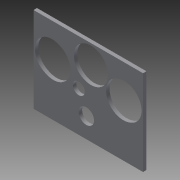
# Autodesk Inventor part: OutlineSketch1
Saved by Autodesk Inventor 2013 (Build 170138000, 138)
## iProperties
Created: 2013-06-03
Part Number: OutlineSketch1
Material: Generic
Document SubType Name: Modeling
Designer: mvarma
Density: 1 g/cm^3
Author: mvarma
Autodesk Inventor part; units mm, degrees
ref_plane "YZ Plane" through (0, 0, 0) normal (1, 0, 0) x (0, 1, 0)
ref_plane "XZ Plane" through (0, 0, 0) normal (0, 1, 0) x (-1, 0, 0)
ref_plane "XY Plane" through (0, 0, 0) normal (0, 0, 1) x (1, 0, 0)
sketch "Sketch1" plane through (0, 0, 0) normal (0, 0, 1) x (1, 0, 0)
  line L0 (0, 0) -> (304.8, 0) construction
  line L1 (304.8, 0) -> (304.8, 50.8) construction
  line L2 (304.8, 50.8) -> (0, 50.8) construction
  line L3 (0, 50.8) -> (0, 0) construction
  circle A0 centre (152.4, 25.4) radius 14.2875
  circle A1 centre (152.4, 25.4) radius 30.48 construction
  circle A2 centre (152.4, 25.4) radius 22.225 construction
  line L4 (152.4, 25.4) -> (138.508178, 62.969727) construction
  circle A3 centre (138.508178, 62.969727) radius 9.525 construction
  circle A4 centre (138.508178, 62.969727) radius 17.78 construction
  circle A5 centre (89.971088, 85.09) radius 31.75 construction
  circle A6 centre (160.978478, 111.345767) radius 31.75
  circle A7 centre (221.970096, 85.09) radius 31.75 construction
  line L5 (0, 50.8) -> (0, 53.34) construction
  line L6 (0, 53.34) -> (304.8, 53.34) construction
  line L7 (304.8, 53.34) -> (304.8, 50.8) construction
  circle A8 centre (138.508178, 62.969727) radius 21.59 construction
  circle A9 centre (152.4, 25.4) radius 46.99 construction
  circle A10 centre (152.4, 25.4) radius 50.8 construction
  arc A11 (84.94082, 79.326416) -> (90.918413, 92.681118) centre (89.971088, 85.09) ccw construction
  circle A12 centre (160.978478, 111.345767) radius 7.65 construction
  arc A13 (221.694578, 92.735037) -> (225.517168, 78.312037) centre (221.970096, 85.09) ccw construction
  circle A14 centre (160.978478, 111.345767) radius 9.1 construction
  circle A15 centre (138.508178, 62.969727) radius 22.9 construction
  line L8 (84.94082, 79.326416) -> (123.450252, 45.716644) construction
  line L9 (168.548316, 110.241211) -> (161.168218, 59.663279) construction
  line L10 (90.918413, 92.681118) -> (89.971088, 85.09) construction
  line L11 (89.971088, 85.09) -> (84.94082, 79.326416) construction
  circle A16 centre (126.19198, 96.27826) radius 3.175 construction
  circle A17 centre (126.19198, 96.27826) radius 7.9375 construction
  line L12 (90.918413, 92.681118) -> (125.209053, 88.401855) construction
  line L13 (132.062639, 90.936044) -> (155.320457, 116.494485) construction
  line L14 (155.320457, 116.494485) -> (160.978478, 111.345767) construction
  line L15 (168.548316, 110.241211) -> (160.978478, 111.345767) construction
  line L16 (138.508178, 62.969727) -> (126.19198, 96.27826) construction
  line L17 (89.971088, 85.09) -> (160.978478, 111.345767) construction
  line L18 (152.4, 25.4) -> (89.971088, 85.09) construction
  line L19 (152.4, 25.4) -> (160.978478, 111.345767) construction
  circle A18 centre (126.19198, 96.27826) radius 9.2075 construction
  circle A19 centre (126.19198, 96.27826) radius 6.1595 construction
  arc A20 (90.918413, 92.681118) -> (84.94082, 79.326416) centre (89.971088, 85.09) ccw construction
  circle A21 centre (160.978478, 111.345767) radius 25.4 construction
  circle A22 centre (221.970096, 85.09) radius 25.4 construction
  line L20 (102.942353, 114.069454) -> (76.999823, 56.110546) construction
  circle A23 centre (89.971088, 85.09) radius 25.4 construction
  line L21 (213.836088, 115.780396) -> (230.104105, 54.399604) construction
  line L22 (54.411088, 146.905767) -> (257.611088, 146.905767)
  line L23 (257.611088, 146.905767) -> (257.611088, -11.844233)
  line L24 (257.611088, -11.844233) -> (54.411088, -11.844233)
  line L25 (54.411088, -11.844233) -> (54.411088, 146.905767)
  circle A24 centre (138.508178, 62.969727) radius 11.1125
  arc A25 (225.312875, 75.445533) -> (221.093638, 95.322667) centre (223.203256, 85.3841) ccw construction
  line L26 (220.753147, 84.734737) -> (228.477303, 60.537683) construction
  line L27 (223.203256, 85.3841) -> (228.477303, 60.537683) construction
  line L28 (220.753147, 84.734737) -> (213.028991, 108.931791) construction
  line L29 (223.203256, 85.3841) -> (217.92921, 110.230517) construction
  arc A26 (212.304851, 111.200264) -> (213.75313, 106.663317) centre (213.028991, 108.931791) ccw construction
  arc A27 (218.423652, 107.901165) -> (217.434768, 112.559869) centre (217.92921, 110.230517) ccw construction
  arc A28 (218.423652, 107.901165) -> (213.75313, 106.663317) centre (228.477303, 60.537683) ccw construction
  arc A29 (217.434768, 112.559869) -> (212.304851, 111.200264) centre (228.477303, 60.537683) ccw construction
  line L30 (213.028991, 108.931791) -> (212.304851, 111.200264) construction
  line L31 (217.92921, 110.230517) -> (217.434768, 112.559869) construction
  arc A30 (221.093638, 95.322667) -> (217.663484, 94.413558) centre (228.477303, 60.537683) ccw construction
  arc A31 (225.312875, 75.445533) -> (223.842809, 75.055915) centre (228.477303, 60.537683) ccw construction
  line L32 (102.635769, 107.180274) -> (91.114923, 84.543355) construction
  line L33 (79.594076, 61.906436) -> (88.801403, 85.578892) construction
  arc A32 (98.871917, 111.470639) -> (97.145543, 107.032054) centre (98.00873, 109.251347) ccw construction
  arc A33 (101.55569, 105.058063) -> (103.715849, 109.302485) centre (102.635769, 107.180274) ccw construction
  arc A34 (101.55569, 105.058063) -> (97.145543, 107.032054) centre (79.594076, 61.906436) ccw construction
  line L34 (98.00873, 109.251347) -> (98.871917, 111.470639) construction
  line L35 (102.635769, 107.180274) -> (103.715849, 109.302485) construction
  arc A35 (103.715849, 109.302485) -> (98.871917, 111.470639) centre (79.594076, 61.906436) ccw construction
  arc A36 (217.663484, 94.413558) -> (223.842809, 75.055915) centre (220.753147, 84.734737) ccw construction
  arc A37 (86.506584, 75.488588) -> (95.723261, 93.598123) centre (91.114923, 84.543355) ccw construction
  line L36 (88.801403, 85.578892) -> (98.00873, 109.251347) construction
  line L37 (91.114923, 84.543355) -> (79.594076, 61.906436) construction
  arc A38 (86.506584, 75.488588) -> (85.118472, 76.10991) centre (79.594076, 61.906436) ccw construction
  arc A39 (95.723261, 93.598123) -> (92.484334, 95.047874) centre (79.594076, 61.906436) ccw construction
  arc A40 (92.484334, 95.047874) -> (85.118472, 76.10991) centre (88.801403, 85.578892) ccw construction
  line L38 (160.978478, 111.345767) -> (138.015112, 122.201357) construction
  line L39 (160.978478, 111.345767) -> (183.941843, 100.490177) construction
  circle A41 centre (138.508178, 62.969727) radius 26.75 construction
  line L40 (221.694578, 92.735037) -> (137.544764, 89.702373) construction
  line L41 (225.517168, 78.312037) -> (150.911337, 39.269007) construction
  line L42 (221.970096, 85.09) -> (221.694578, 92.735037) construction
  line L43 (221.970096, 85.09) -> (225.517168, 78.312037) construction
  line L44 (138.508178, 62.969727) -> (137.544764, 89.702373) construction
  line L45 (138.508178, 62.969727) -> (150.911337, 39.269007) construction
  arc A42 (225.517168, 78.312037) -> (221.694578, 92.735037) centre (221.970096, 85.09) ccw construction
  arc A43 (225.517168, 78.312037) -> (224.776319, 77.973286) centre (221.970096, 85.09) ccw construction
  line L46 (138.508178, 62.969727) -> (221.970096, 85.09) construction
  circle A44 centre (88.801403, 85.578892) radius 31.75
  circle A45 centre (91.114923, 84.543355) radius 31.75
  line L47 (98.871917, 111.470639) -> (100.310562, 115.16946) construction
  line L48 (103.715849, 109.302485) -> (105.515981, 112.839504) construction
  arc A46 (105.515981, 112.839504) -> (100.310562, 115.16946) centre (79.594076, 61.906436) ccw
  circle A47 centre (220.753147, 84.734737) radius 31.75
  circle A48 centre (223.203256, 85.3841) radius 31.75
  line L49 (212.304851, 111.200264) -> (211.097951, 114.981054) construction
  line L50 (217.434768, 112.559869) -> (216.610698, 116.442121) construction
  arc A49 (216.610698, 116.442121) -> (211.097951, 114.981054) centre (228.477303, 60.537683) ccw
  point P0 (215.46289, 109.642317)
  point P1 (100.3481, 108.273564)
  dimension "d114" = 63.5
  dimension "d115" = 63.5
  dimension "d122" = 63.5
  dimension "d123" = 63.5
  dimension "d1" = 50.8
  dimension "d2" = 28.575
  dimension "d3" = 25.4
  dimension "d4" = 152.4
  dimension "d7" = 60.96
  dimension "d8" = 44.45
  dimension "d9" = 19.05
  dimension "d10" = 35.56
  dimension "d11" = 40.0558
  dimension "d12" = 63.5
  dimension "d13" = 63.5
  dimension "d14" = 63.5
  dimension "d15" = 2.54
  dimension "d16" = 304.8
  dimension "d17" = 43.18
  dimension "d18" = 93.98
  dimension "d19" = 101.6
  dimension "d21" = 15.3
  dimension "d22" = 15.3
  dimension "d24" = 18.2
  dimension "d29" = 45.8
  dimension "d30" = 146
  dimension "d31" = 6.35
  dimension "d32" = 15.875
  dimension "d33" = 146
  dimension "d35" = 18.415
  dimension "d37" = 12.319
  dimension "d40" = 50.8
  dimension "d41" = 50.8
  dimension "d42" = 17
  dimension "d43" = 17
  dimension "d44" = 50.8
  dimension "d53" = 203.2
  dimension "d54" = 158.75
  dimension "d55" = 35.56
  dimension "d56" = 35.56
  dimension "d57" = 22.225
  dimension "d67" = 25.4
  dimension "d68" = 25.4
  dimension "d69" = 2.86
  dimension "d70" = 25.4
  dimension "d71" = 25.4
  dimension "d72" = 4.7625
  dimension "d75" = 2.86
  dimension "d80" = 4.7625
  dimension "d82" = 4.7625
  dimension "d83" = 50.8
  dimension "d84" = 50.8
  dimension "d85" = 10.16
  dimension "d97" = 48.41875
  dimension "d99" = 20.32
  dimension "d101" = 25.4
  dimension "d102" = 25.4
  dimension "d103" = 10.16
  dimension "d105" = 17
  dimension "d106" = 17
  dimension "d107" = 53.5
  dimension "d108" = 154.44
  dimension "d109" = 7.65
  dimension "d111" = 86.34349
  dimension "d112" = 12.7801
  dimension "d113" = 12.7801
  dimension "d116" = 57.15
  constraints: 104 end point, 67 point on circle, 46 centre point, 38 coincident, 18 tangent, 14 collinear, 14 point on line, 9 perpendicular, 7 parallel, 2 horizontal, 2 midpoint, 1 equal radius, 15 other
  measures "d1" distance of L1.end L0.end
  measures "d2" diameter of A0
  measures "d3" distance from line of L0 A0.centre
  measures "d4" distance from line of L3 A0.centre
  measures "d7" diameter of A1
  measures "d8" diameter of A2
  measures "d9" diameter of A3
  measures "d10" diameter of A4
  measures "d11" distance of L4.start L4.end
  measures "d12" diameter of A5
  measures "d13" diameter of A6
  measures "d14" diameter of A7
  measures "d15" distance of L2.end L5.end
  measures "d16" distance of L0.end L0.start
  measures "d17" diameter of A8
  measures "d18" diameter of A9
  measures "d19" diameter of A10
  measures "d21" diameter of A11
  measures "d22" diameter of A12
  measures "d24" diameter of A14
  measures "d29" diameter of A15
  measures "d30" angle of L11 L10
  measures "d31" diameter of A16
  measures "d32" diameter of A17
  measures "d33" angle of L15 L14
  measures "d35" diameter of A18
  measures "d37" diameter of A19
  measures "d40" diameter of A21
  measures "d41" diameter of A22
  measures "d42" angle of L10 L20
  measures "d43" angle of L11 L20
  measures "d44" diameter of A23
  measures "d53" distance of L23.end L24.end
  measures "d54" distance of L22.end L23.end
  measures "d55" distance from line of L25 A5.centre
  measures "d56" distance from line of L22 A6.centre
  measures "d57" diameter of A24
  measures "d67" distance of L26.start L26.end
  measures "d68" distance of L27.start L26.end
  measures "d69" angle of L21 L26
  measures "d70" distance of L26.start L28.end
  measures "d71" distance of L27.start L29.end
  measures "d72" diameter of A26
  measures "d75" angle of L20 L32
  measures "d80" diameter of A32
  measures "d82" diameter of A33
  measures "d83" distance of L33.start L36.end
  measures "d84" distance of L32.start L33.start
  measures "d85" radius of A25
  measures "d97" radius of A34
  measures "d99" diameter of A37
  measures "d101" distance of L33.start L33.end
  measures "d102" distance of L32.end L33.start
  measures "d103" radius of A40
  measures "d105" angle of L38 L14
  measures "d106" angle of L39 L15
  measures "d107" diameter of A41
  measures "d108" angle of L42 L43
  measures "d109" radius of A13
  measures "d111" distance of L44.start L42.start
  measures "d112" angle of L21 L42
  measures "d113" angle of L21 L43
  measures "d116" radius of A46
sketch "Sketch1 outline for Extrusion3" plane through (0, 0, 0) normal (0, 0, 1) x (1, 0, 0)
  line L0 (54.411088, 146.905767) -> (257.611088, 146.905767)
  line L1 (54.411088, -11.844233) -> (54.411088, 146.905767)
  line L2 (257.611088, 146.905767) -> (257.611088, -11.844233)
  line L3 (257.611088, -11.844233) -> (54.411088, -11.844233)
  circle A0 centre (152.4, 25.4) radius 14.2875
  circle A1 centre (138.508178, 62.969727) radius 11.1125
  arc A2 (122.864923, 84.543355) -> (102.91909, 114.017482) centre (91.114923, 84.543355) ccw
  arc A3 (102.91909, 114.017482) -> (76.997235, 56.104765) centre (88.801403, 85.578892) ccw
  arc A4 (76.997235, 56.104765) -> (122.864923, 84.543355) centre (91.114923, 84.543355) ccw
  arc A5 (254.953256, 85.3841) -> (213.850676, 115.725355) centre (223.203256, 85.3841) ccw
  arc A6 (213.850676, 115.725355) -> (230.105727, 54.393482) centre (220.753147, 84.734737) ccw
  arc A7 (230.105727, 54.393482) -> (254.953256, 85.3841) centre (223.203256, 85.3841) ccw
  circle A8 centre (160.978478, 111.345767) radius 31.75
extrude "Extrusion3" add sketch "Sketch1 outline for Extrusion3" along normal blind 6.35
equation "\"d2\" = BearingLargeOD"
equation "\"d7\" = Gear48tPD"
equation "\"d8\" = Gear35tPD"
equation "\"d9\" = Gear15tPD"
equation "\"d10\" = Gear28tPD"
equation "\"d11\" = 0.5 * Gear48tPD + 0.5 * Gear15tPD + MeshingClearance"
equation "\"d12\" = CimOD"
equation "\"d13\" = CimOD"
equation "\"d14\" = CimOD"
equation "\"d17\" = Gear28tPD + ClearanceDiameter"
equation "\"d18\" = WheelOD"
equation "\"d19\" = WheelClearance"
equation "\"Pulley48tPD\" = 45.8"
equation "\"Pulley19tPD\" = 18.2"
equation "\"Pulley16tPD\" = 15.3"
equation "\"Gear15tPD\" = 19.05"
equation "\"Gear35tPD\" = 44.45"
equation "\"Gear48tPD\" = 60.96"
equation "\"Gear28tPD\" = 35.56"
equation "\"BearingLargeOD\" = 28.575"
equation "\"BearingSmallOD\" = 22.225"
equation "\"MeshingClearance\" = 0.0508"
equation "\"CimOD\" = 63.5"
equation "\"WheelOD\" = 93.98"
equation "\"ClearanceDiameter\" = 7.62"
equation "\"WheelClearance\" = 101.6"
equation "\"TensioningBearingID\" = 6.35"
equation "\"TensioningBearingOD\" = 15.875"
equation "\"SpingClipClearance\" = 8.89"
equation "\"Pi\" = 79.79645"
equation "\"Pulley56tPD\" = 53.5"
equation "\"BearingXLargeOD\" = 34.925"
body "Solid3"
